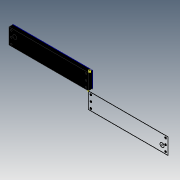
# Autodesk Inventor part: gripsupport
Saved by Autodesk Inventor 2015 (Build 190159000, 159)
## iProperties
Created: 2014-08-31
Part Number: gripsupport
Material: Generic
Document SubType Name: Modeling
Designer: shohei
Density: 1 g/cm^3
Appearance: Default
Mass: 80 g
Surface Area: 208 cm^2
Volume: 80 cm^3
Author: shohei
Autodesk Inventor part; units mm, degrees
ref_plane "YZ Plane" through (0, 0, 0) normal (1, 0, 0) x (0, 1, 0)
ref_plane "XZ Plane" through (0, 0, 0) normal (0, 1, 0) x (-1, 0, 0)
ref_plane "XY Plane" through (0, 0, 0) normal (0, 0, 1) x (1, 0, 0)
sketch "Block1" plane through (0, 0, 0) normal (0, 0, 1) x (1, 0, 0)
  line L0 (0.22, -40.22) -> (-200.22, -40.22)
  line L1 (-200.22, -40.22) -> (-200.22, 0.22)
  line L2 (-200.22, 0.22) -> (0.22, 0.22)
  line L3 (0.22, 0.22) -> (0.22, -40.22)
  circle A0 centre (-5.9987, -35) radius 2.22
  circle A1 centre (-5.9987, -20) radius 2.22
  circle A2 centre (-5.9987, -5) radius 2.22
  circle A3 centre (-185, -25) radius 5.22
  circle A4 centre (-194.0013, -35) radius 2.22
  circle A5 centre (-194.0013, -5) radius 2.22
  circle A6 centre (-194.0013, -20) radius 2.22
  point P0 (-106.5385, -20.3846)
sketch "Sketch1" plane through (0, 0, 0) normal (0, 1, 0) x (-1, 0, 0)
  line L0 (0, 0) -> (200, 0)
  line L1 (200, 0) -> (200, 40)
  line L2 (200, 40) -> (0, 40)
  line L3 (0, 40) -> (0, 0)
  circle A0 centre (5.9987, 5) radius 2
  line L4 (5.9987, -4.5949) -> (5.9987, 47.4768)
  circle A1 centre (5.9987, 35) radius 2
  circle A2 centre (5.9987, 20) radius 2
  line L5 (100, 57.9252) -> (100, -15.7167)
  circle A3 centre (194.0013, 5) radius 2
  circle A4 centre (194.0013, 35) radius 2
  circle A5 centre (194.0013, 20) radius 2
  circle A6 centre (185, 25) radius 5
  dimension "d0" = 200
  dimension "d1" = 40
  dimension "d4" = 4
  dimension "d5" = 4
  dimension "d6" = 5
  dimension "d7" = 5
  dimension "d8" = 4
  dimension "d9" = 20
  dimension "d10" = 100
  dimension "d13" = 10
  dimension "d14" = 15
  dimension "d15" = 15
  constraints: 12 end point, 7 centre point, 3 symmetric about line, 2 parallel, 2 point on line, 2 vertical, 1 horizontal, 1 perpendicular, 3 other
  measures "d0" distance of L1.end L2.end
  measures "d1" distance of L0.end L1.end
  measures "d4" diameter of A0
  measures "d5" diameter of A1
  measures "d6" distance from line of L2 A1.centre
  measures "d7" distance from line of L0 A0.centre
  measures "d8" diameter of A2
  measures "d9" distance from line of L2 A2.centre
  measures "d10" distance between parallel lines of L3 L5
  measures "d13" diameter of A6
  measures "d14" distance from line of L2 A6.centre
  measures "d15" distance from line of L1 A6.centre
extrude "Extrusion3" add sketch "Sketch1" along normal blind 10 contours L3 L2 L4 A1 A2 A0 L0 | L4 A0 A2 A1 L2 L5 L0 | L5 L2 L1 L0
sketch "Sketch2" plane through (0, 10, 0) normal (0, 1, 0) x (1, 0, 0)
  circle A0 centre (-185, -25) radius 5 projected
  circle A1 centre (-194.0013, -20) radius 2 projected
  circle A2 centre (-194.0013, -35) radius 2 projected
  circle A3 centre (-194.0013, -5) radius 2 projected
  circle A4 centre (-5.9987, -20) radius 2 projected
  circle A5 centre (-5.9987, -35) radius 2 projected
  circle A6 centre (-5.9987, -5) radius 2 projected
  line L0 (0, 0) -> (-200, 0) projected
  line L1 (-200, 0) -> (-200, -40) projected
  line L2 (-200, -40) -> (0, -40) projected
  line L3 (0, -40) -> (0, 0) projected
  line L4 (0.22, -40.22) -> (-200.22, -40.22)
  line L5 (-200.22, -40.22) -> (-200.22, 0.22)
  line L6 (-200.22, 0.22) -> (0.22, 0.22)
  line L7 (0.22, 0.22) -> (0.22, -40.22)
  circle A7 centre (-5.9987, -35) radius 2.22
  circle A8 centre (-5.9987, -20) radius 2.22
  circle A9 centre (-5.9987, -5) radius 2.22
  circle A10 centre (-185, -25) radius 5.22
  circle A11 centre (-194.0013, -35) radius 2.22
  circle A12 centre (-194.0013, -5) radius 2.22
  circle A13 centre (-194.0013, -20) radius 2.22
  constraints: 3 perpendicular, 7 other
sketch "DXF" plane through (0, 0, 0) normal (0, 1, 0) x (-1, 0, 0)
  line L0 (0.22, -40.22) -> (-200.22, -40.22)
  line L1 (-200.22, -40.22) -> (-200.22, 0.22)
  line L2 (-200.22, 0.22) -> (0.22, 0.22)
  line L3 (0.22, 0.22) -> (0.22, -40.22)
  circle A0 centre (-5.9987, -35) radius 2.22
  circle A1 centre (-5.9987, -20) radius 2.22
  circle A2 centre (-5.9987, -5) radius 2.22
  circle A3 centre (-185, -25) radius 5.22
  circle A4 centre (-194.0013, -35) radius 2.22
  circle A5 centre (-194.0013, -5) radius 2.22
  circle A6 centre (-194.0013, -20) radius 2.22
  point P0 (0, 0)
body "Solid3"
